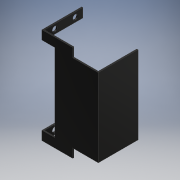
# Autodesk Inventor part: Shoulder Plate
Saved by Autodesk Inventor 2017 (Build 210142000, 142)
## iProperties
Created: 2018-10-14
Part Number: Shoulder Plate
Material: Generic
Document SubType Name: Modeling
Designer: Cameron
Density: 1 g/cm^3
Appearance: Glossy - Black
Author: Cameron
Autodesk Inventor part; units mm, degrees
ref_plane "YZ Plane" through (0, 0, 0) normal (1, 0, 0) x (0, 1, 0)
ref_plane "XZ Plane" through (0, 0, 0) normal (0, 1, 0) x (-1, 0, 0)
ref_plane "XY Plane" through (0, 0, 0) normal (0, 0, 1) x (1, 0, 0)
sketch "Sketch1" plane through (0, 0, 0) normal (0, 1, 0) x (-1, 0, 0)
  line L0 (0, 0) -> (44, 0)
  line L1 (44, -75) -> (20, -75)
  line L2 (0, -75) -> (0, -7)
  line L3 (44, 0) -> (44, -7)
  line L4 (44, -7) -> (34, -7)
  line L5 (34, -7) -> (34, -68)
  line L6 (34, -68) -> (44, -68)
  line L7 (44, 0) -> (44, -7)
  line L8 (44, -68) -> (44, -75)
  line L9 (0, 0) -> (20, 0)
  line L10 (20, 0) -> (20, -7)
  line L11 (20, -7) -> (0, -7)
  line L12 (20, -68) -> (20, -75)
  line L13 (20, -68) -> (0, -68)
  dimension "d0" = 44
  dimension "d1" = 75
  dimension "d2" = 7
  dimension "d3" = 10
  dimension "d4" = 61
  dimension "d5" = 20
  constraints: 28 end point, 7 perpendicular, 4 point on line, 3 parallel, 2 vertical, 1 horizontal
  measures "d0" distance of L1.start L2.start
  measures "d1" distance of L0.end L1.start
  measures "d2" distance of L0.end L3.end
  measures "d3" distance of L3.end L4.end
  measures "d4" distance of L4.end L5.end
  measures "d5" distance of L0.start L9.end
extrude "Extrusion1" add sketch "Sketch1" along normal blind 1
sketch "Sketch2" plane through (0, 1, 0) normal (0, 1, 0) x (1, 0, 0)
  line L0 (0, 68) -> (-20, 68) projected
  line L1 (-20, 75) -> (-44, 75) projected
  line L2 (-34, 7) -> (-44, 7) projected
  line L3 (-44, 0) -> (-43, 0)
  line L4 (-43, 0) -> (-43, 7)
  line L5 (-43, 7) -> (-44, 7)
  line L6 (-44, 7) -> (-44, 0)
  line L7 (-44, 68) -> (-43, 68)
  line L8 (-43, 68) -> (-43, 75)
  line L9 (-43, 75) -> (-44, 75)
  line L10 (-44, 75) -> (-44, 68)
  line L11 (0, 7) -> (-1, 7)
  line L12 (-1, 7) -> (-1, 68)
  line L13 (-1, 68) -> (0, 68)
  line L14 (0, 68) -> (0, 7)
  point P0 (0, 0)
  dimension "d8" = 1
  dimension "d9" = 1
  dimension "d10" = 1
  constraints: 24 end point, 6 parallel, 3 horizontal, 3 perpendicular, 3 point on line
  measures "d8" distance of L5.end L4.end
  measures "d9" distance of L9.end L8.end
  measures "d10" distance of L12.end L13.end
extrude "Extrusion2" add sketch "Sketch2" along normal blind 30
sketch "Sketch3" plane through (-44, 0, -7) normal (-1, 0, 0) x (0, 0, 1)
  line L0 (0, 31) -> (7, 31) projected
  line L1 (3.5, 31) -> (3.5, 25)
  line L2 (3.5, 25) -> (3.5, 9)
  circle A0 centre (3.5, 25) radius 2
  circle A1 centre (3.5, 9) radius 2
  dimension "d13" = 6
  dimension "d14" = 16
  dimension "d15" = 4
  dimension "d16" = 4
  constraints: 4 end point, 2 centre point, 2 coincident, 1 midpoint, 1 point on line, 1 vertical
  measures "d13" distance of L1.start L1.end
  measures "d14" distance of L1.end L2.end
  measures "d15" diameter of A0
  measures "d16" diameter of A1
extrude "Extrusion3" cut sketch "Sketch3" against normal blind 30
sketch "Sketch4" plane through (-44, 0, -75) normal (-1, 0, 0) x (0, 0, 1)
  line L0 (7, 31) -> (0, 31) projected
  line L1 (3.5, 31) -> (3.5, 25)
  line L2 (3.5, 25) -> (3.5, 9)
  circle A0 centre (3.5, 25) radius 2
  circle A1 centre (3.5, 9) radius 2
  point P0 (75, 0)
  dimension "d19" = 6
  dimension "d20" = 16
  dimension "d21" = 4
  dimension "d22" = 4
  constraints: 4 end point, 2 centre point, 2 coincident, 1 midpoint, 1 point on line, 1 vertical
  measures "d19" distance of L1.start L1.end
  measures "d20" distance of L1.end L2.end
  measures "d21" diameter of A0
  measures "d22" diameter of A1
extrude "Extrusion4" cut sketch "Sketch4" against normal blind 30
body "Solid1"
